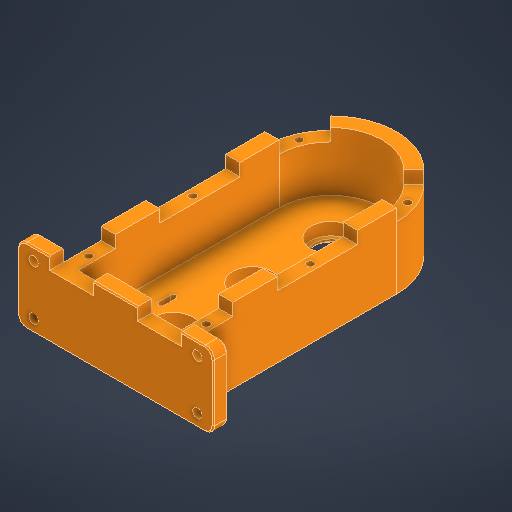
# Autodesk Inventor part: Segmento inferior
Saved by Autodesk Inventor 2026 (Build 300175050, 175E)
## iProperties
Created: 2025-07-26
Part Number: Segmento inferior
Material: Plastico PETG
Document SubType Name: Modeling
Designer: bello
Density: 1.27 g/cm^3
Appearance: Naranja
Author: bello
Autodesk Inventor part; units mm, degrees
ref_plane "YZ Plane" through (0, 0, 0) normal (1, 0, 0) x (0, 1, 0)
ref_plane "XZ Plane" through (0, 0, 0) normal (0, 1, 0) x (-1, 0, 0)
ref_plane "XY Plane" through (0, 0, 0) normal (0, 0, 1) x (1, 0, 0)
sketch "Boceto1" plane through (0, 0, 0) normal (0, 1, 0) x (-1, 0, 0)
  line L0 (-55, 0) -> (0, 0)
  line L1 (0, 0) -> (0, -8)
  line L2 (0, -8) -> (-18, -8)
  line L3 (-18, -8) -> (-18, -121)
  line L4 (-55, 0) -> (-110, 0)
  line L5 (-110, 0) -> (-110, -8)
  line L6 (-110, -8) -> (-92, -8)
  line L7 (-92, -8) -> (-92, -121)
  circle A0 centre (-55, -121) radius 9
  circle A1 centre (-55, -77) radius 9
  line L8 (0, 74.4962) -> (0, 12.0402)
  line L9 (-55, -25.5) -> (-55, -32.5) construction
  line L10 (-66.1, -25.5) -> (-66.1, -32.5)
  line L11 (-43.9, -32.5) -> (-43.9, -25.5)
  arc A2 (-43.9, -25.5) -> (-66.1, -25.5) centre (-55, -25.5) ccw
  arc A3 (-66.1, -32.5) -> (-43.9, -32.5) centre (-55, -32.5) ccw
  line L12 (-39.5, -10) -> (-39.5, -17) construction
  line L13 (-41.05, -10) -> (-41.05, -17)
  line L14 (-37.95, -17) -> (-37.95, -10)
  arc A4 (-37.95, -10) -> (-41.05, -10) centre (-39.5, -10) ccw
  arc A5 (-41.05, -17) -> (-37.95, -17) centre (-39.5, -17) ccw
  line L15 (-55, -21.4) -> (-55, -36.6)
  line L16 (-61.9919, -29) -> (-48.019, -29)
  line L17 (-39.5, -48) -> (-39.5, -41) construction
  line L18 (-41.05, -48) -> (-41.05, -41)
  line L19 (-37.95, -41) -> (-37.95, -48)
  arc A6 (-41.05, -48) -> (-37.95, -48) centre (-39.5, -48) ccw
  arc A7 (-37.95, -41) -> (-41.05, -41) centre (-39.5, -41) ccw
  line L20 (-70.5, -10) -> (-70.5, -17) construction
  line L21 (-68.95, -10) -> (-68.95, -17)
  line L22 (-72.05, -17) -> (-72.05, -10)
  arc A8 (-68.95, -10) -> (-72.05, -10) centre (-70.5, -10) ccw
  arc A9 (-72.05, -17) -> (-68.95, -17) centre (-70.5, -17) ccw
  arc A10 (-68.95, -41) -> (-72.05, -41) centre (-70.5, -41) ccw
  line L23 (-68.95, -48) -> (-68.95, -41)
  line L24 (-70.5, -48) -> (-70.5, -41) construction
  arc A11 (-72.05, -48) -> (-68.95, -48) centre (-70.5, -48) ccw
  line L25 (-72.05, -41) -> (-72.05, -48)
  arc A12 (-92, -121) -> (-18, -121) centre (-55, -121) ccw
  point P0 (-55, -29)
  point P1 (-39.5, -13.5)
  point P2 (-39.5, -44.5)
  point P3 (-70.5, -13.5)
  point P4 (-70.5, -44.5)
  point P5 (-55, -158)
  dimension "d2" = 8
  dimension "d3" = 18
  dimension "d12" = 18
  dimension "d13" = 18
  dimension "d38" = 8
  dimension "d41" = 22.2
  dimension "d42" = 7
  dimension "d45" = 7
  dimension "d46" = 3.1
  dimension "d47" = 15.5
  dimension "d48" = 15.5
  dimension "d128" = 74
  dimension "d129" = 113
  dimension "d136" = 158
  dimension "d137" = 44
  dimension "d138" = 44.5
  dimension "d139" = 7
  constraints: 62 end point, 23 point on circle, 21 symmetric about line, 13 centre point, 8 tangent, 4 vertical, 3 horizontal, 3 perpendicular, 2 midpoint, 2 parallel, 1 coincident, 1 point on line, 6 other
  measures "d2" distance of L0.end L1.end
  measures "d3" distance of L1.end L2.end
  measures "d12" diameter of A0
  measures "d13" diameter of A1
  measures "d38" distance of L5.start L5.end
  measures "d41" distance between parallel lines of L10 L11
  measures "d42" distance of L11.start L11.end
  measures "d45" distance of L14.start L14.end
  measures "d46" distance between parallel lines of L13 L14
  measures "d47" distance between parallel lines of L9 L12
  measures "d48" horizontal distance of L9.start L12.start
  measures "d128" diameter of A12
  measures "d129" distance of L6.end L7.end
  measures "d136" distance from line of L4 point (-55, -158)
  measures "d137" distance of A1.centre A0.centre
  measures "d138" distance of L9.end A1.centre
  measures "d139" distance of L9.start L9.end
extrude "Extrusión1" add sketch "Boceto1" along normal blind 42
sketch "Boceto2" plane through (0, 42, 0) normal (0, 1, 0) x (1, 0, 0)
  line L0 (84, 8) -> (26, 8)
  line L1 (0, 0) -> (110, 0) projected
  line L2 (18, 121) -> (18, 8) projected
  line L3 (92, 8) -> (92, 121) projected
  line L4 (26, 8) -> (26, 121)
  line L5 (84, 8) -> (84, 121)
  circle A0 centre (55, 121) radius 9 projected
  arc A1 (84, 121) -> (26, 121) centre (55, 121) ccw
  point P0 (0, 0)
  dimension "d23" = 8
  dimension "d61" = 58
  dimension "d62" = 8
  dimension "d63" = 8
  dimension "d130" = 58
  constraints: 6 end point, 2 point on circle, 2 vertical, 1 centre point, 1 coincident
  measures "d23" distance between parallel lines of L1 L0
  measures "d61" distance of L0.start L0.end
  measures "d62" distance between parallel lines of L4 L2
  measures "d63" distance from line of L3 L0.start
  measures "d130" diameter of A1
extrude "Extrusión2" cut sketch "Boceto2" against normal blind 33 contours L0 L4 A1 L5 | A0
sketch "Boceto3" plane through (0, 9, 0) normal (0, 1, 0) x (1, 0, 0)
  circle A0 centre (55, 77) radius 9 projected
  circle A1 centre (55, 77) radius 11.1
  circle A2 centre (55, 121) radius 9 projected
  circle A3 centre (55, 121) radius 11.1
  point P0 (0, 0)
  dimension "d51" = 22.2
  constraints: 2 centre point, 2 coincident, 1 equal radius
  measures "d51" diameter of A1
extrude "Extrusión3" cut sketch "Boceto3" against normal blind 7
sketch "Boceto4" plane through (0, 42, 0) normal (0, 1, 0) x (1, 0, 0)
  line L0 (18, 0) -> (18, 29)
  line L1 (18, 0) -> (42.6, 0)
  line L2 (42.6, 0) -> (42.6, 8)
  line L3 (18, 29) -> (26, 29)
  line L4 (26, 29) -> (26, 8)
  line L5 (26, 8) -> (42.6, 8)
  line L6 (55, -21.8553) -> (55, 186.6483)
  line L7 (18, 54) -> (26, 54)
  line L8 (26, 99) -> (18, 99)
  line L9 (18, 54) -> (18, 99)
  line L10 (26, 54) -> (26, 99)
  line L11 (26, 8) -> (26, 121) projected
  line L12 (18, 121) -> (26, 121)
  line L13 (49.3086, 121) -> (59.8366, 121)
  arc A0 (34.4939, 141.5061) -> (26, 121) centre (55.8313, 120.6557) ccw
  arc A1 (28.837, 147.163) -> (18, 121) centre (55, 121) ccw
  line L14 (55, 121) -> (34.4939, 141.5061)
  line L15 (34.4939, 141.5061) -> (28.837, 147.163)
  line L16 (92, 0) -> (92, 29)
  line L17 (92, 0) -> (67.4, 0)
  line L18 (67.4, 0) -> (67.4, 8)
  line L19 (92, 29) -> (84, 29)
  line L20 (84, 29) -> (84, 8)
  line L21 (84, 8) -> (67.4, 8)
  line L22 (92, 54) -> (84, 54)
  line L23 (84, 99) -> (92, 99)
  line L24 (92, 54) -> (92, 99)
  line L25 (84, 54) -> (84, 99)
  line L26 (84, 8) -> (84, 121)
  line L27 (92, 121) -> (84, 121)
  arc A2 (84, 121) -> (75.5061, 141.5061) centre (54.1687, 120.6557) ccw
  arc A3 (92, 121) -> (81.163, 147.163) centre (55, 121) ccw
  line L28 (55, 121) -> (75.5061, 141.5061)
  line L29 (75.5061, 141.5061) -> (81.163, 147.163)
  point P0 (84, 8)
  dimension "d54" = 29
  dimension "d55" = 24.6
  dimension "d56" = 25
  dimension "d57" = 45
  dimension "d132" = 45
  constraints: 58 end point, 15 symmetric about line, 8 point on circle, 4 centre point, 3 horizontal, 2 vertical, 1 collinear, 3 other
  measures "d54" distance of L0.start L0.end
  measures "d55" distance of L0.start L1.end
  measures "d56" distance between parallel lines of L3 L7
  measures "d57" distance between parallel lines of L8 L7
  measures "d132" angle of L13 L14
extrude "Extrusión4" cut sketch "Boceto4" against normal blind 7
sketch "Boceto5" plane through (0, 0, 0) normal (0, 0, 1) x (1, 0, 0)
  circle A0 centre (9, 35) radius 2.6
  line L0 (0, 42) -> (18, 42) projected
  line L1 (0, 0) -> (0, 42) projected
  circle A1 centre (9, 7) radius 2.6
  circle A2 centre (101, 35) radius 2.6
  circle A3 centre (101, 7) radius 2.6
  line L2 (0, 0) -> (110, 0) projected
  line L3 (110, 0) -> (110, 42) projected
  line L4 (42.6, 42) -> (110, 42) projected
  point P0 (92, 42)
  dimension "d75" = 5.2
  dimension "d76" = 7
  dimension "d77" = 9
  dimension "d115" = 7
  dimension "d116" = 9
  dimension "d117" = 7
  dimension "d118" = 9
  dimension "d119" = 7
  dimension "d120" = 9
  constraints: 4 centre point
  measures "d75" diameter of A0
  measures "d76" distance from line of L0 A0.centre
  measures "d77" distance from line of L1 A0.centre
  measures "d115" distance from line of L2 A1.centre
  measures "d116" distance from line of L1 A1.centre
  measures "d117" distance from line of L2 A3.centre
  measures "d118" distance from line of L3 A3.centre
  measures "d119" distance from line of L4 A2.centre
  measures "d120" distance from line of L3 A2.centre
extrude "Extrusión5" cut sketch "Boceto5" against normal through all
sketch "Boceto6" plane through (110, 0, -8) normal (0, 0, -1) x (-1, 0, 0)
  circle A0 centre (9, 35) radius 2.6 projected
  line L0 (11.396, 39.15) -> (13.792, 35)
  line L1 (13.792, 35) -> (11.396, 30.85)
  line L2 (11.396, 30.85) -> (6.604, 30.85)
  line L3 (6.604, 30.85) -> (4.208, 35)
  line L4 (4.208, 35) -> (6.604, 39.15)
  line L5 (6.604, 39.15) -> (11.396, 39.15)
  circle A1 centre (101, 35) radius 2.6
  line L6 (98.604, 39.15) -> (96.208, 35)
  line L7 (96.208, 35) -> (98.604, 30.85)
  line L8 (98.604, 30.85) -> (103.396, 30.85)
  line L9 (103.396, 30.85) -> (105.792, 35)
  line L10 (105.792, 35) -> (103.396, 39.15)
  line L11 (103.396, 39.15) -> (98.604, 39.15)
  circle A2 centre (9, 7) radius 2.6 projected
  line L12 (13.792, 7) -> (11.396, 2.85)
  line L13 (11.396, 2.85) -> (6.604, 2.85)
  line L14 (6.604, 2.85) -> (4.208, 7)
  line L15 (4.208, 7) -> (6.604, 11.15)
  line L16 (6.604, 11.15) -> (11.396, 11.15)
  line L17 (11.396, 11.15) -> (13.792, 7)
  circle A3 centre (101, 7) radius 2.6 projected
  line L18 (105.792, 7) -> (103.396, 2.85)
  line L19 (103.396, 2.85) -> (98.604, 2.85)
  line L20 (98.604, 2.85) -> (96.208, 7)
  line L21 (96.208, 7) -> (98.604, 11.15)
  line L22 (98.604, 11.15) -> (103.396, 11.15)
  line L23 (103.396, 11.15) -> (105.792, 7)
  point P0 (110, 0)
  point P1 (9, 2.85)
  point P2 (9, 11.15)
  dimension "d80" = 8.3
  dimension "d121" = 8.3
  dimension "d122" = 8.3
  dimension "d123" = 8.3
  constraints: 48 end point, 4 coincident, 2 midpoint, 1 centre point, 39 other
  measures "d80" distance between parallel lines of L2 L5
  measures "d121" distance between parallel lines of L8 L11
  measures "d122" distance of point (9, 2.85) point (9, 11.15)
  measures "d123" distance between parallel lines of L19 L22
extrude "Extrusión6" cut sketch "Boceto6" against normal blind 3.5 contours L0 L1 L2 L3 L4 L5 | L11 L10 L9 L8 L7 L6 | A2 | L12 L13 L14 L15 L16 L17 | L18 L19 L20 L21 L22 L23
fillet "Empalme1" radius 5 4 edges at (110, 42, -4) (110, 0, -4) (0, 42, -4) (0, 0, -4)
chamfer "Chaflán1" distance 0.7 angle 45 42 edges at (64, 0, -77) (64, 0, -121) (43.9, 0, -29) (55, 0, -43.6) (66.1, 0, -29) (55, 0, -14.4) (37.95, 0, -44.5) (39.5, 0, -49.55) (41.05, 0, -44.5) (39.5, 0, -39.45) (68.95, 0, -44.5) (70.5, 0, -49.55) (72.05, 0, -44.5) (70.5, 0, -39.45) (68.95, 0, -13.5) (70.5, 0, -18.55) (72.05, 0, -13.5) (70.5, 0, -8.45) (37.95, 0, -13.5) (39.5, 0, -18.55) (41.05, 0, -13.5) (39.5, 0, -8.45) (98.5, 0, -8) (108.5355, 1.4645, -8) (110, 21, -8) (108.5355, 40.5355, -8) (98.5, 42, -8) (11.5, 0, -8) (1.4645, 1.4645, -8) (0, 21, -8) (1.4645, 40.5355, -8) (11.5, 42, -8) (55, 0, 0) (108.5355, 1.4645, 0) (110, 21, 0) (108.5355, 40.5355, 0) (98.5, 42, 0) (11.5, 42, 0) (55, 42, 0) (1.4645, 1.4645, 0) (0, 21, 0) (1.4645, 40.5355, 0)
sketch "Boceto7" plane through (0, 35, 0) normal (0, 1, 0) x (1, 0, 0)
  circle A0 centre (22, 76.5) radius 2.05
  circle A1 centre (22, 18) radius 2.05
  line L0 (26, 29) -> (26, 8) projected
  line L1 (26, 99) -> (26, 54) projected
  line L2 (26, 99) -> (26, 54) projected
  line L3 (18, 29) -> (26, 29) projected
  line L4 (18, 99) -> (26, 99) projected
  circle A2 centre (55, 77) radius 11.1 projected
  line L5 (55, -15.2989) -> (55, 167.3429)
  circle A3 centre (55, 121) radius 9 projected
  circle A4 centre (55, 121) radius 33
  circle A5 centre (24.512, 133.6286) radius 2.05
  line L6 (24.512, 133.6286) -> (55, 121)
  line L7 (47.9496, 121) -> (62.3852, 121)
  circle A6 centre (88, 76.5) radius 2.05
  circle A7 centre (88, 18) radius 2.05
  circle A8 centre (85.488, 133.6286) radius 2.05
  line L8 (85.488, 133.6286) -> (55, 121)
  point P0 (0, 0)
  dimension "d133" = 66
  dimension "d87" = 4.1
  dimension "d88" = 4
  dimension "d89" = 4
  dimension "d94" = 11
  dimension "d95" = 22.5
  dimension "d134" = 22.5
  dimension "d135" = 4.1
  constraints: 8 end point, 6 centre point, 3 symmetric about line, 1 coincident, 1 equal radius, 1 horizontal, 1 vertical, 6 other
  measures "d87" diameter of A0
  measures "d88" distance from line of L0 A1.centre
  measures "d89" distance from line of L1 A0.centre
  measures "d94" distance from line of L3 A1.centre
  measures "d95" distance from line of A0.centre L4
  measures "d134" angle of L7 L6
  measures "d135" diameter of A5
extrude "Extrusión7" cut sketch "Boceto7" against normal blind 5.8 contours A0 | A1 | A8 L8 A4 | A4 A8 | A5 A4 | A4 L6 A5 | L8 A8 A4 | A4 A5 L6 | A6 | A7
equation "\"d10\" = Altura"
equation "\"Altura\" = 42"
